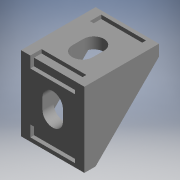
# Autodesk Inventor part: 14056_m
Saved by Autodesk Inventor 2017.3 (Build 213256000, 256)
## iProperties
Part Number: 14056_m
Material: Generic
Catalog Web Link: www.cadenas.de
Description: 14056, 14051, 14053, 14052, 14054_m-2 Hole Inside Corner Brackets
Vendor: 8020
Document SubType Name: Modeling
Designer: partserver
Manufacturer: 8020
Mass: 2.09215 g
Surface Area: 21.6591 cm^2
Volume: 2.09215 cm^3
Density: 1 g/cm^3
Appearance: PSOLRGB-175-175-175
Category: PARTsolutions
Company: 8020
Title: 14056
Author: Cadenas PARTsolutions
Comments: 2 Hole Inside Corner Brackets
PSOL_IDENT_0: {$CADENAS_DATA\23d-libs\8020\metric\joining_plates\14056_m.prj},186 {VTYP=3D},{NB=14056_m},{LINA=140
PSOL_IDENT_1: 56},{NN=14056, 14051, 14053, 14052, 14054_m},{DATE=31.07.2020 09:21:28},{GEOMDATE=09.09.2015 07:48:2
PSOL_IDENT_2: 3},{VERSION=},{LINEID=10},{WBVAR=FIN,D},{WBNUMERIC=}  {NB=14056_m},{LINA=14056},{KT=DUMMY},{PN=14056
PSOL_IDENT_3: },{MAT=Die Cast Zinc},{FIN=1},{A=20.00},{B=17.00},{C=5.50},{D=},{D1= '','None','5','5.00' },{D2=0.00
PSOL_IDENT_4: },{T=2.00},{W=.013},{CC=5-20, 6-10, 6-25}
NB: 14056_m
NN: 14056, 14051, 14053, 14052, 14054_m
NT: 2 Hole Inside Corner Brackets
NBSYN: $PN._m
LINA: 14056
CATALOG: 80/20
PN: 14056
MAT: Die Cast Zinc
FIN: Natural
A: 20
B: 17
C: 5.5
T: 2
W: .013
CC: 5-20, 6-10, 6-25
SUPPLIER: 8020
ARTICLENO: 14056_m
BOMINFO: 14056
CREATOR: CADENAS GmbH
Autodesk Inventor part; units mm, degrees
ref_plane "YZ Plane" through (0, 0, 0) normal (1, 0, 0) x (0, 1, 0)
ref_plane "XZ Plane" through (0, 0, 0) normal (0, 1, 0) x (-1, 0, 0)
ref_plane "XY Plane" through (0, 0, 0) normal (0, 0, 1) x (1, 0, 0)
sketch "Sketch_1" plane through (0, 0, 0) normal (1, 0, 0) x (0, 1, 0)
  line L0 (0, 20) -> (0, 0)
  line L1 (0, 0) -> (20, 0)
  line L2 (20, 0) -> (20, 3)
  line L3 (20, 3) -> (3, 20)
  line L4 (3, 20) -> (0, 20)
  constraints: 10 end point
extrude "Extrusion1" add sketch "Sketch_1" along normal mid plane 17
sketch "Sketch_2" plane through (0, 0, 0) normal (1, 0, 0) x (0, 1, 0)
  line L0 (3, 20) -> (3, 3.5)
  arc A0 (3, 3.5) -> (3.5, 3) centre (3.5, 3.5) ccw
  line L1 (3.5, 3) -> (20, 3)
  line L2 (20, 3) -> (3, 20)
  constraints: 6 end point, 2 point on circle, 1 centre point
extrude "Extrusion2" cut sketch "Sketch_2" along normal mid plane 13
sketch "Sketch_3" plane through (0, 0, 0) normal (1, 0, 0) x (0, 1, 0)
  line L0 (0, 3) -> (0, 0)
  line L1 (0, 0) -> (3, 0)
  line L2 (3, 0) -> (3, 1)
  line L3 (3, 1) -> (1, 1)
  line L4 (1, 1) -> (1, 3)
  line L5 (1, 3) -> (0, 3)
  constraints: 12 end point
extrude "Extrusion3" cut sketch "Sketch_3" along normal mid plane 12
sketch "Sketch_4" plane through (0, 0, 0) normal (1, 0, 0) x (0, 1, 0)
  line L0 (0, 19) -> (0, 16)
  line L1 (0, 16) -> (1, 16)
  line L2 (1, 16) -> (1, 19)
  line L3 (1, 19) -> (0, 19)
  constraints: 8 end point
extrude "Extrusion4" cut sketch "Sketch_4" along normal mid plane 12
sketch "Sketch_5" plane through (0, 0, 0) normal (1, 0, 0) x (0, 1, 0)
  line L0 (16, 1) -> (16, 0)
  line L1 (16, 0) -> (19, 0)
  line L2 (19, 0) -> (19, 1)
  line L3 (19, 1) -> (16, 1)
  constraints: 8 end point
extrude "Extrusion5" cut sketch "Sketch_5" along normal mid plane 12
sketch "Sketch_10" plane through (0, 0, 0) normal (0, 1, 0) x (-1, 0, 0)
  line L0 (2.75, 8) -> (2.75, 11)
  arc A0 (2.75, 11) -> (-2.75, 11) centre (0, 11) ccw
  line L1 (-2.75, 11) -> (-2.75, 8)
  arc A1 (-2.75, 8) -> (2.75, 8) centre (0, 8) ccw
  constraints: 4 end point, 4 point on circle, 2 centre point
extrude "Extrusion6" cut sketch "Sketch_10" along normal blind 5
sketch "Sketch_11" plane through (0, 0, 0) normal (0, 0, 1) x (1, 0, 0)
  arc A0 (-2.75, 8) -> (2.75, 8) centre (0, 8) ccw
  line L0 (2.75, 8) -> (2.75, 11)
  arc A1 (2.75, 11) -> (-2.75, 11) centre (0, 11) ccw
  line L1 (-2.75, 11) -> (-2.75, 8)
  constraints: 4 end point, 4 point on circle, 2 centre point
extrude "Extrusion7" cut sketch "Sketch_11" along normal blind 5
body "Solid1"
